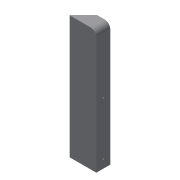
# Autodesk Inventor part: komatex_senzor
Saved by Autodesk Inventor 2015 (Build 190159000, 159)
## iProperties
Created: 2015-01-04
Part Number: komatex_senzor
Material: Generic
Document SubType Name: Modeling
Designer: Turboslimak
Density: 1 g/cm^3
Appearance: Default
Author: Turboslimak
Autodesk Inventor part; units mm, degrees
ref_plane "YZ Plane" through (0, 0, 0) normal (1, 0, 0) x (0, 1, 0)
ref_plane "XZ Plane" through (0, 0, 0) normal (0, 1, 0) x (-1, 0, 0)
ref_plane "XY Plane" through (0, 0, 0) normal (0, 0, 1) x (1, 0, 0)
sketch "Sketch1" plane through (0, 0, 0) normal (0, 1, 0) x (-1, 0, 0)
  line L0 (9.5, -44) -> (-9.5, -44)
  line L1 (-9.5, -44) -> (-9.5, 44)
  line L2 (-9.5, 44) -> (9.5, 44)
  line L3 (9.5, 44) -> (9.5, -44)
  line L4 (9.5, -44) -> (-9.5, 44) construction
  line L5 (-9.5, -44) -> (9.5, 44) construction
  point P0 (0, 0)
  dimension "d0" = 19
  dimension "d1" = 88
  constraints: 12 end point, 2 midpoint, 2 parallel, 1 horizontal, 1 perpendicular
  measures "d0" distance of L1.end L2.end
  measures "d1" distance of L0.end L1.end
extrude "Extrusion1" add sketch "Sketch1" along normal blind 10
fillet "Fillet1" radius 4 1 edges at (9.5, 5, 44)
chamfer "Chamfer1" distance 9.5 angle 45 1 edges at (-9.5, 10, 0)
sketch "Sketch2" plane through (9.5, 0, -44) normal (1, 0, 0) x (0, 0, -1)
  line L0 (0, 0) -> (-50, 0)
  line L1 (-50, 0) -> (-50, 5)
  line L2 (-50, 5) -> (0, 5)
  line L3 (0, 5) -> (0, 0)
  line L4 (-6, 5.5) -> (-44, 5.5)
  line L5 (-44, 5.5) -> (-44, 4.5)
  line L6 (-44, 4.5) -> (-6, 4.5)
  line L7 (-6, 4.5) -> (-6, 5.5)
  line L8 (-6, 5.5) -> (-44, 4.5) construction
  line L9 (-44, 5.5) -> (-6, 4.5) construction
  circle A0 centre (-44, 5) radius 0.5
  circle A1 centre (-6, 5) radius 0.5
  point P0 (-44, 0)
  point P1 (-25, 5)
  dimension "d8" = 50
  dimension "d9" = 5
  dimension "d10" = 38
  dimension "d11" = 1
  dimension "d12" = 1
  dimension "d13" = 1
  constraints: 20 end point, 5 midpoint, 4 parallel, 2 centre point, 2 horizontal, 2 perpendicular
  measures "d8" distance of L1.end L2.end
  measures "d9" distance of L0.end L1.end
  measures "d10" distance of L6.end L5.end
  measures "d11" distance of L5.end L4.end
  measures "d12" diameter of A0
  measures "d13" diameter of A1
extrude "Extrusion2" cut sketch "Sketch2" against normal blind 2 contours A1 L7 L2 | L2 L7 A1 | A0 L5 L2 | L2 L5 A0 | L7 A1 L2 | L2 A1 L7 | L5 A0 L2 | L2 A0 L5
body "Solid1"
